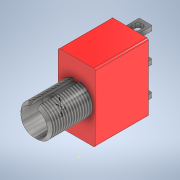
# Autodesk Inventor part: switch
Saved by Autodesk Inventor 2022.2 (Build 262287000, 287)
## iProperties
Created: 2022-01-24
Part Number: switch
Material: Stainless Steel
Document SubType Name: Modeling
Designer: hugof
Density: 8 g/cm^3
Appearance: Semi-Polished
Author: hugof
Autodesk Inventor part; units mm, degrees
ref_plane "YZ Plane" through (0, 0, 0) normal (1, 0, 0) x (0, 1, 0)
ref_plane "XZ Plane" through (0, 0, 0) normal (0, 1, 0) x (-1, 0, 0)
ref_plane "XY Plane" through (0, 0, 0) normal (0, 0, 1) x (1, 0, 0)
sketch "Sketch1" plane through (0, 0, 0) normal (0, 0, 1) x (1, 0, 0)
  line L0 (0, 0) -> (-6.96, 0)
  line L1 (-6.96, 0) -> (-6.96, 12.8)
  line L2 (-6.96, 12.8) -> (0, 12.8)
  line L3 (0, 12.8) -> (0, 0)
  dimension "d0" = 6.96
  dimension "d1" = 12.8
  constraints: 8 end point, 2 perpendicular, 1 horizontal, 1 vertical
  measures "d0" distance of L0.start L0.end
  measures "d1" distance of L0.end L1.end
sketch "Sketch1 outline for Extrusion1" plane through (0, 0, 0) normal (0, 0, 1) x (1, 0, 0)
  line L0 (0, 0) -> (0, 12.8)
  line L1 (-6.96, 0) -> (0, 0)
  line L2 (-6.96, 12.8) -> (-6.96, 0)
  line L3 (0, 12.8) -> (-6.96, 12.8)
extrude "Extrusion1" add sketch "Sketch1 outline for Extrusion1" along normal blind 10
sketch "Sketch3" plane through (0, 0, 0) normal (0, 0, -1) x (-1, 0, 0)
  line L0 (4.713973, 12.26) -> (2.246027, 12.26)
  line L1 (2.246027, 12.26) -> (2.246027, 11.44)
  line L2 (2.246027, 11.44) -> (4.713973, 11.44)
  line L3 (4.713973, 11.44) -> (4.713973, 12.26)
  line L4 (0, 12.8) -> (6.96, 12.8)
  line L5 (6.96, 0) -> (0, 0)
  line L6 (4.713973, 11.44) -> (6.96, 11.44)
  line L7 (6.96, 12.8) -> (6.96, 0)
  line L8 (2.246027, 11.44) -> (0, 11.44)
  line L9 (0, 0) -> (0, 12.8)
  line L10 (0, 6.4) -> (6.96, 6.4)
  line L11 (0, 12.8) -> (6.96, 12.8)
  line L12 (6.96, 12.8) -> (6.96, 6.4)
  line L13 (6.96, 6.4) -> (6.96, 0)
  line L14 (4.713973, 12.26) -> (4.713973, 11.44)
  line L15 (2.246027, 12.26) -> (2.246027, 11.44)
  line L16 (4.713973, 6.4) -> (4.713973, 6.81)
  line L17 (4.713973, 6.81) -> (2.246027, 6.81)
  line L18 (2.246027, 6.81) -> (2.246027, 6.4)
  line L19 (4.713973, 0.54) -> (2.246027, 0.54)
  line L20 (2.246027, 0.54) -> (2.246027, 1.36)
  line L21 (2.246027, 1.36) -> (4.713973, 1.36)
  line L22 (4.713973, 1.36) -> (4.713973, 0.54)
  line L23 (4.713973, 6.4) -> (4.713973, 5.99)
  line L24 (4.713973, 5.99) -> (2.246027, 5.99)
  line L25 (2.246027, 5.99) -> (2.246027, 6.4)
  dimension "d4" = 0.82
  dimension "d6" = 11.44
  dimension "d7" = 0.41
  constraints: 42 end point, 6 symmetric about line, 5 collinear, 5 perpendicular, 5 point on line, 2 midpoint, 1 horizontal, 1 vertical
  measures "d4" distance of L2.end L0.start
  measures "d6" distance between parallel lines of L5 L2
  measures "d7" distance of L16.start L16.end
sketch "Sketch3 outline for Extrusion2" plane through (0, 0, 0) normal (0, 0, -1) x (-1, 0, 0)
  line L0 (2.246027, 1.36) -> (2.246027, 0.54)
  line L1 (4.713973, 1.36) -> (2.246027, 1.36)
  line L2 (4.713973, 0.54) -> (4.713973, 1.36)
  line L3 (2.246027, 0.54) -> (4.713973, 0.54)
  line L4 (4.713973, 6.81) -> (2.246027, 6.81)
  line L5 (2.246027, 6.81) -> (2.246027, 5.99)
  line L6 (2.246027, 5.99) -> (4.713973, 5.99)
  line L7 (4.713973, 5.99) -> (4.713973, 6.81)
  line L8 (4.713973, 12.26) -> (2.246027, 12.26)
  line L9 (4.713973, 11.44) -> (4.713973, 12.26)
  line L10 (2.246027, 11.44) -> (4.713973, 11.44)
  line L11 (2.246027, 12.26) -> (2.246027, 11.44)
extrude "Extrusion2" add sketch "Sketch3 outline for Extrusion2" along normal blind 3
sketch "Sketch4" plane through (-4.713973, 12.26, 0) normal (0, 1, 0) x (1, 0, 0)
  line L0 (1.967945, 0.5) -> (1.967945, 2.3)
  line L1 (1.967945, 2.3) -> (0.5, 2.3)
  line L2 (0.5, 2.3) -> (0.5, 0.5)
  line L3 (0.5, 0.5) -> (1.967945, 0.5)
  line L4 (2.467945, 0) -> (2.467945, 3)
  line L5 (0, 0) -> (0, 3)
  line L6 (0, 3) -> (2.467945, 3)
  point P0 (4.713973, 0)
  dimension "d10" = 0.5
  dimension "d11" = 0.5
  dimension "d12" = 1.8
  dimension "d13" = 0.7
  constraints: 8 end point, 3 perpendicular
  measures "d10" distance between parallel lines of L4 L0
  measures "d11" distance between parallel lines of L5 L2
  measures "d12" distance of L0.start L0.end
  measures "d13" distance between parallel lines of L6 L1
sketch "Sketch4 outline for Extrusion3" plane through (-4.713973, 12.26, 0) normal (0, 1, 0) x (1, 0, 0)
  line L0 (1.967945, 0.5) -> (1.967945, 2.3)
  line L1 (0.5, 0.5) -> (1.967945, 0.5)
  line L2 (0.5, 2.3) -> (0.5, 0.5)
  line L3 (1.967945, 2.3) -> (0.5, 2.3)
extrude "Extrusion3" cut sketch "Sketch4 outline for Extrusion3" against normal through all
fillet "Fillet1" radius 0.5 12 edges at (-4.214, 11.85, -2.3) (-2.746, 11.85, -2.3) (-4.214, 11.85, -0.5) (-2.746, 11.85, -0.5) (-4.214, 6.4, -0.5) (-2.746, 6.4, -0.5) (-2.746, 6.4, -2.3) (-4.214, 0.95, -2.3) (-4.214, 6.4, -2.3) (-2.746, 0.95, -0.5) (-4.214, 0.95, -0.5) (-2.746, 0.95, -2.3)
fillet "Fillet2" radius 0.2 6 edges at (-4.714, 11.85, -3) (-4.714, 6.4, -3) (-4.714, 0.95, -3) (-2.246, 0.95, -3) (-2.246, 6.4, -3) (-2.246, 11.85, -3)
fillet "Fillet3" radius 0.3 4 edges at (0, 0, 5) (-6.96, 0, 5) (0, 12.8, 5) (-6.96, 12.8, 5)
sketch "Sketch5" plane through (0, 0, 10) normal (0, 0, 1) x (1, 0, 0)
  circle A0 centre (-3.48, 6.4) radius 3
  line L0 (-6.96, 12.5) -> (-6.96, 0.3) projected
  line L1 (-3.48, 6.4) -> (-3.48, 12.8)
  line L2 (-0.3, 12.8) -> (-6.66, 12.8) projected
  line L3 (-6.66, 12.8) -> (-3.48, 12.8)
  line L4 (-3.48, 12.8) -> (-0.3, 12.8)
  line L5 (-6.96, 6.4) -> (-3.48, 6.4)
  line L6 (-3.48, 6.4) -> (0, 6.4)
  line L7 (0, 0.3) -> (0, 12.5) projected
  line L8 (-3.48, 6.4) -> (-3.48, 0)
  line L9 (-6.66, 0) -> (-0.3, 0) projected
  point P0 (0, 0)
  dimension "d19" = 6
  constraints: 12 end point, 4 midpoint, 3 horizontal, 2 collinear, 1 centre point, 1 point on line
  measures "d19" diameter of A0
sketch "Sketch5 outline for Extrusion4" plane through (0, 0, 10) normal (0, 0, 1) x (1, 0, 0)
  circle A0 centre (-3.48, 6.4) radius 3
extrude "Extrusion4" add sketch "Sketch5 outline for Extrusion4" along normal blind 8
sketch "Sketch6" plane through (-3.48, 6.4, 18) normal (0, 0, 1) x (1, 0, 0)
  circle A0 centre (0, 0) radius 3 projected
  circle A1 centre (0, 0) radius 2.5
  point P0 (3.48, -6.4)
  dimension "d41" = 5
  constraints: 1 centre point, 1 coincident
  measures "d41" diameter of A1
sketch "Sketch6 outline for Extrusion5" plane through (-3.48, 6.4, 18) normal (0, 0, 1) x (1, 0, 0)
  circle A0 centre (0, 0) radius 2.5
extrude "Extrusion5" cut sketch "Sketch6 outline for Extrusion5" against normal blind 4
thread "Thread1" size "M3x0.5" class "6g" standard "ISO Metric profile" full length
chamfer "Chamfer1" distance 0.5 angle 45 1 edges at (-6.48, 6.4, 18)
sketch "Sketch10" plane through (-3.48, 6.4, 14) normal (0, 0, 1) x (1, 0, 0)
  circle A0 centre (0, 0) radius 2.5
  line L0 (0.625, 2.420615) -> (0.625, 2.934174)
  circle A1 centre (0, 0) radius 3
  line L1 (-0.625, 2.420615) -> (-0.625, 2.934174)
  arc A2 (0.625, 2.934174) -> (-0.625, 2.934174) centre (0, 0) ccw
  arc A3 (0.625, 2.420615) -> (-0.625, 2.420615) centre (0, 0.520779) ccw
  point P0 (3.48, -6.4)
  constraints: 8 point on circle, 4 end point, 2 centre point, 1 concentric, 1 parallel, 1 vertical
sketch "Sketch10 outline for Extrusion6" plane through (-3.48, 6.4, 14) normal (0, 0, 1) x (1, 0, 0)
  line L0 (-0.625, 2.934174) -> (-0.625, 2.420615)
  arc A0 (0.625, 2.934174) -> (-0.625, 2.934174) centre (0, 0) ccw
  line L1 (0.625, 2.420615) -> (0.625, 2.934174)
  arc A1 (-0.625, 2.420615) -> (0.625, 2.420615) centre (0, 0) cw
extrude "Extrusion6" cut sketch "Sketch10 outline for Extrusion6" along normal mid plane 8
sketch "Sketch11" plane through (-3.48, 6.4, 14) normal (0, 0, 1) x (1, 0, 0)
  circle A0 centre (0, 0) radius 1
  point P0 (3.48, -6.4)
  constraints: 1 centre point
sketch "Sketch11 outline for Extrusion7" plane through (-3.48, 6.4, 14) normal (0, 0, 1) x (1, 0, 0)
  circle A0 centre (0, 0) radius 1
extrude "Extrusion7" cut sketch "Sketch11 outline for Extrusion7" against normal blind 1
sketch "Sketch13" plane through (-3.48, 6.4, 13) normal (0, 0, 1) x (1, 0, 0)
  circle A0 centre (0, 0) radius 0.95
  line L0 (0.949991, -0.004201) -> (-0.949991, 0.004201)
  circle A1 centre (0, 0) radius 2
  circle A2 centre (0, 0) radius 1.5
  point P0 (3.48, -6.4)
  dimension "d39" = 1.9
  dimension "d44" = 3
  constraints: 3 centre point, 2 coincident, 2 end point, 2 point on circle, 1 midpoint
  measures "d39" diameter of A0
  measures "d44" diameter of A2
sketch "Sketch13 outline for Revolution2" plane through (-3.48, 6.4, 13) normal (0, 0, 1) x (1, 0, 0)
  line L0 (-0.949991, 0.004201) -> (0.949991, -0.004201)
  arc A0 (0.949991, -0.004201) -> (-0.949991, 0.004201) centre (0, 0) ccw
revolve "Revolution2" add sketch "Sketch13 outline for Revolution2" angle 360 about axis through (-2.530009, 6.395799, 13) along (-0.9999902, 0.0044216, 0)
body "Solid1"
